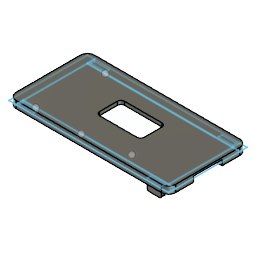
lidwithhole (Autodesk Fusion 360 design; units mm, degrees)
part number: 2026-04-18-08-50-46-334
Autodesk Fusion 360 part; units mm, degrees
note: some values were not read from the file. Chosen so that the rebuilt part matches the saved one: which face or edge a step refers to; which pieces of a blend or face edit are solid. Set by a fixed rule: which sketch regions a step uses.
sketch "Sketch1" plane through (0, 0, 0) normal (0, 0, 1) x (1, 0, 0)
  line L0 (24.6565, 31.9846) -> (24.6565, -4.0154)
  line L1 (24.6565, -4.0154) -> (-24.3435, -4.0154)
  line L2 (14.6565, 31.9846) -> (-46.8435, 31.9846)
  line L3 (-56.8435, 31.9846) -> (24.6565, 31.9846)
  line L4 (-56.8435, 35.9846) -> (-60.8435, 35.9846)
  line L5 (-56.8435, 31.9846) -> (24.6565, 31.9846)
  line L6 (-56.8435, -4.0154) -> (-56.8435, 31.9846)
  line L7 (24.6565, -4.0154) -> (-56.8435, -4.0154)
  line L8 (-56.8435, 35.9846) -> (-56.8435, 31.9846)
  line L9 (-56.8435, -8.0154) -> (-56.8435, -4.0154)
  line L10 (-56.8435, -4.0154) -> (-49.8435, -4.0154)
  line L11 (-56.8435, -8.0154) -> (-56.8435, 35.9846)
  line L12 (-60.8435, -8.0154) -> (-56.8435, -8.0154)
  line L13 (-60.8435, 35.9846) -> (-60.8435, -8.0154)
  line L14 (24.6565, 31.9846) -> (28.6565, 31.9846)
  line L15 (28.6565, 31.9846) -> (28.6565, 35.9846)
  line L16 (28.6565, 35.9846) -> (24.6565, 35.9846)
  line L17 (24.6565, 35.9846) -> (24.6565, 31.9846)
  line L18 (24.6565, 35.9846) -> (-56.8435, 35.9846)
  line L19 (-56.8435, 35.9846) -> (-56.8435, 31.9846)
  line L20 (-56.8435, 31.9846) -> (24.6565, 31.9846)
  line L21 (24.6565, 31.9846) -> (24.6565, 35.9846)
  line L22 (28.6565, 31.9846) -> (24.6565, 31.9846)
  line L23 (24.6565, 31.9846) -> (24.6565, -4.0154)
  line L24 (24.6565, -4.0154) -> (28.6565, -4.0154)
  line L25 (28.6565, -4.0154) -> (28.6565, 31.9846)
  line L26 (28.6565, -4.0154) -> (-56.8435, -4.0154)
  line L27 (-56.8435, -4.0154) -> (-56.8435, -8.0154)
  line L28 (-56.8435, -8.0154) -> (28.6565, -8.0154)
  line L29 (28.6565, -8.0154) -> (28.6565, -4.0154)
  line L30 (-55.8435, 34.9846) -> (-47.8435, 34.9846)
  line L31 (-47.8435, 34.9846) -> (-47.8435, 32.9846)
  line L32 (-47.8435, 32.9846) -> (-55.8435, 32.9846)
  line L33 (-55.8435, 32.9846) -> (-55.8435, 34.9846)
  line L34 (23.6565, 34.9846) -> (15.6565, 34.9846)
  line L35 (15.6565, 34.9846) -> (15.6565, 32.9846)
  line L36 (15.6565, 32.9846) -> (23.6565, 32.9846)
  line L37 (23.6565, 32.9846) -> (23.6565, 34.9846)
  line L38 (23.6565, -5.0154) -> (15.6565, -5.0154)
  line L39 (15.6565, -5.0154) -> (15.6565, -7.0154)
  line L40 (15.6565, -7.0154) -> (23.6565, -7.0154)
  line L41 (23.6565, -7.0154) -> (23.6565, -5.0154)
  line L42 (-55.8435, -5.0154) -> (-47.8435, -5.0154)
  line L43 (-47.8435, -5.0154) -> (-47.8435, -7.0154)
  line L44 (-47.8435, -7.0154) -> (-55.8435, -7.0154)
  line L45 (-55.8435, -7.0154) -> (-55.8435, -5.0154)
  dimension "d73" = 36
  dimension "d75" = 4
  dimension "d78" = 4
  dimension "d81" = 4
  dimension "d82" = 44
  dimension "d93" = 4
  dimension "d94" = 4
  dimension "d97" = 8
  dimension "d98" = 2
  dimension "d99" = 5
  dimension "d100" = 1
  dimension "d101" = 8
  dimension "d102" = 2
  dimension "d103" = 8
  dimension "d104" = 2
  dimension "d105" = 8
  dimension "d106" = 2
  dimension "d107" = 5
  dimension "d108" = 1
  dimension "d109" = 1
  dimension "d110" = 5
  dimension "d111" = 5
  dimension "d112" = 1
  constraint horizontal L3
  constraint vertical L0
  constraint vertical L6
  constraint horizontal L5
  constraint vertical L8
  constraint horizontal L2
  constraint coincident L2.start L5
  constraint horizontal L4
  constraint vertical L13
  constraint horizontal L12
  constraint vertical L11
  constraint horizontal L14
  constraint vertical L15
  constraint horizontal L16
  constraint vertical L17
  constraint horizontal L18
  constraint vertical L19
  constraint horizontal L20
  constraint vertical L21
  constraint horizontal L22
  constraint vertical L23
  constraint horizontal L24
  constraint vertical L25
  constraint horizontal L26
  constraint vertical L27
  constraint horizontal L28
  constraint vertical L29
  constraint horizontal L30
  constraint vertical L31
  constraint horizontal L32
  constraint vertical L33
  constraint horizontal L34
  constraint vertical L35
  constraint horizontal L36
  constraint vertical L37
  constraint horizontal L38
  constraint vertical L39
  constraint horizontal L40
  constraint vertical L41
  constraint horizontal L42
  constraint vertical L43
  constraint horizontal L44
  constraint vertical L45
  measures "d73" distance of L3.start L6.start
  measures "d75" distance of L6.start L9.start
  measures "d78" distance of L3.start L4.start
  measures "d81" distance of L4.end L4.start
  measures "d82" distance of L4.start L9.start
  measures "d93" distance of L0.start L14.end
  measures "d94" distance of L0.start L16.end
  measures "d97" distance of L30.start L30.end
  measures "d98" distance of L30.start L32.end
  measures "d99" distance of L13 L33
  measures "d100" distance of L18 L30
  measures "d101" distance of L34.start L34.end
  measures "d102" distance of L34.start L36.end
  measures "d103" distance of L38.start L38.end
  measures "d104" distance of L38.start L40.end
  measures "d105" distance of L42.start L42.end
  measures "d106" distance of L42.start L44.end
  measures "d107" distance of L13 L45
  measures "d108" distance of L26 L42
  measures "d109" distance of L26 L38
  measures "d110" distance of L29 L41
  measures "d111" distance of L15 L37
  measures "d112" distance of L18 L34
sketch "Sketch2" plane through (-60.8435, 0, 0) normal (-1, 0, 0) x (0, -1, 0)
  line L0 (-32.4846, 0) -> (-32.4846, -4)
  line L1 (-32.4846, -4) -> (3.0154, -4)
  line L2 (3.0154, -4) -> (3.0154, 0)
  line L3 (3.0154, 0) -> (-32.4846, 0)
  line L4 (-22.4846, -4) -> (-7.4846, -4)
  line L5 (-7.4846, -4) -> (-7.4846, -1)
  line L6 (-7.4846, -1) -> (-22.4846, -1)
  line L7 (-22.4846, -1) -> (-22.4846, -4)
  dimension "d59" = 15
  dimension "d60" = 3
  dimension "d61" = 10
  constraint horizontal L4
  constraint vertical L5
  constraint horizontal L6
  constraint vertical L7
  constraint coincident L1 L4.start
  measures "d59" distance of L4.start L4.end
  measures "d60" distance of L4.start L6.end
  measures "d61" distance of L0 L7
extrude "Extrude7" add sketch "Sketch1" along normal blind 2 contours L0 L14 L22 L23 L24 L25 L26 | L0 L1 L2 L3 L5 L6 L7 L10 L11 L20 L23 L26 | L14 L15 L16 L17 L21 L22 | L2 L3 L5 L8 L11 L17 L18 L19 L20 L21 | L1 L7 L9 L10 L11 L24 L26 L27 L28 L29 | L4 L6 L8 L9 L11 L12 L13 L19 L27 | L30 L31 L32 L33 | L34 L35 L36 L37 | L38 L39 L40 L41 | L42 L43 L44 L45 makes body 1
fillet "Fillet7" radius 4 14 edges at (-60.8435, -8.0154, 1) (-58.8435, -8.0154, 0) (-58.8435, -8.0154, 2) (28.6565, -8.0154, 1) (28.6565, -6.0154, 0) (28.6565, -6.0154, 2) (28.6565, 35.9846, 1) (28.6565, 33.9846, 0) (28.6565, 33.9846, 2) (26.6565, 35.9846, 0) (26.6565, 35.9846, 2) (-60.8435, 35.9846, 1) (-58.8435, 35.9846, 0) (-58.8435, 35.9846, 2) on bodies 1
sketch "Sketch3" plane through (0, 0, 2) normal (0, 0, 1) x (-1, 0, 0)
  arc A0 (-24.6565, 8.0154) -> (-28.6565, 4.0154) centre (-24.6565, 4.0154) ccw
  line L0 (-28.6565, 4.0154) -> (-28.6565, -31.9846)
  arc A1 (-28.6565, -31.9846) -> (-24.6565, -35.9846) centre (-24.6565, -31.9846) ccw
  line L1 (-24.6565, -35.9846) -> (56.8435, -35.9846)
  arc A2 (56.8435, -35.9846) -> (60.8435, -31.9846) centre (56.8435, -31.9846) ccw
  line L2 (60.8435, -31.9846) -> (60.8435, 4.0154)
  arc A3 (60.8435, 4.0154) -> (56.8435, 8.0154) centre (56.8435, 4.0154) ccw
  line L3 (56.8435, 8.0154) -> (-24.6565, 8.0154)
  line L4 (28.0435, -21.9846) -> (3.0435, -21.9846)
  line L5 (3.0435, -21.9846) -> (3.0435, -7.9846)
  line L6 (3.0435, -7.9846) -> (28.0435, -7.9846)
  line L7 (28.0435, -7.9846) -> (28.0435, -21.9846)
  line L8 (60.8435, -35.9846) -> (60.8435, 8.0154)
  line L9 (56.8435, 8.0154) -> (-28.6565, 8.0154)
  dimension "d121" = 32.8
  dimension "d122" = 25
  dimension "d124" = 14
  dimension "d146" = 14
  constraint horizontal L4
  constraint vertical L5
  constraint horizontal L6
  constraint vertical L7
  measures "d121" distance of L7 L8
  measures "d122" distance of L5 L7
  measures "d124" distance of L4 L6
  measures "d146" distance of L1 L4
extrude "Extrude10" cut sketch "Sketch3" against normal blind 8 contours L4 L5 L6 L7 bodies 1
fillet "Fillet9" radius 2 4 edges at (-28.0435, 21.9846, 1) (-3.0435, 21.9846, 1) (-3.0435, 7.9846, 1) (-28.0435, 7.9846, 1) on bodies 1
extrude "Extrude11" add sketch "Sketch1" against normal blind 2 contours L0 L14 L22 L23 L24 L25 L26 | L14 L15 L16 L17 L21 L22 | L2 L3 L5 L8 L11 L17 L18 L19 L20 L21 | L1 L7 L9 L10 L11 L24 L26 L27 L28 L29 | L4 L6 L8 L9 L11 L12 L13 L19 L27 bodies 1
fillet "Fillet10" radius 4 4 edges at (-60.8435, -8.0154, -1) (-60.8435, 35.9846, -1) (28.6565, -8.0154, -1) (28.6565, 35.9846, -1) on bodies 1
extrude "Extrude12" add 3 faces at (-53.1768, -6.3487, 0) (18.3232, -6.3487, 0) (-53.1768, 33.6513, 0) along direction (0, 0, -1) blind 6 on bodies 1 bodies 1
fillet "Fillet11" radius 1 6 edges at (-55.8435, -6.0154, -6) (-47.8435, -6.0154, -6) (-55.8435, 33.9846, -6) (-47.8435, 33.9846, -6) (15.6565, -6.0154, -6) (23.6565, -6.0154, -6) on bodies 1
sketch "Sketch4" plane through (28.6565, 0, 0) normal (1, 0, 0) x (0, 1, 0)
  line L0 (31.9846, -2) -> (31.9846, 2)
  line L1 (31.9846, 2) -> (-4.0154, 2)
  line L2 (-4.0154, 2) -> (-4.0154, -2)
  line L3 (-4.0154, -2) -> (31.9846, -2)
  line L4 (5.9846, -2) -> (21.9846, -2)
  line L5 (21.9846, -2) -> (21.9846, 1)
  line L6 (21.9846, 1) -> (5.9846, 1)
  line L7 (5.9846, 1) -> (5.9846, -2)
  dimension "d137" = 3
  dimension "d138" = 10
  dimension "d139" = 10
  constraint horizontal L4
  constraint vertical L5
  constraint horizontal L6
  constraint vertical L7
  constraint coincident L3 L4.start
  measures "d137" distance of L4.start L6.end
  measures "d138" distance of L2 L7
  measures "d139" distance of L0 L5
extrude "Extrude13" cut sketch "Sketch4" against normal blind 8 contours L3 L4 L5 L6 L7 bodies 1
fillet "Fillet12" radius 1 2 edges at (20.6565, 5.9846, 0.5) (20.6565, 21.9846, 0.5) on bodies 1
fillet "Fillet13" radius 1 2 edges at (24.6565, 21.9846, -1) (24.6565, 5.9846, -1) on bodies 1
delete_face "DeleteFace2" 1 faces at (-52.8435, 34.9846, -3.3333) on bodies 1
extrude "Extrude14" add 1 faces at (18.3232, 33.6513, 0) along direction (0, 0, -1) blind 6 on bodies 1 bodies 1
fillet "Fillet14" radius 1 2 edges at (23.6565, 33.9846, -6) (15.6565, 33.9846, -6) on bodies 1
delete_face "DeleteFace3" 1 faces at (-52.8435, -7.0154, -3.3333) on bodies 1
extrude "Extrude15" add sketch "Sketch1" against normal blind 6 separate body contours L30 L31 L32 L33 makes body 2
fillet "Fillet15" radius 1 2 edges at (-55.8435, 33.9846, -6) (-47.8435, 33.9846, -6) on bodies 2
